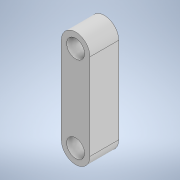
# Autodesk Inventor part: GearLock
Saved by Autodesk Inventor 2021 (Build 250183000, 183)
## iProperties
Created: 2021-03-28
Part Number: GearLock
Material: Generic
Document SubType Name: Modeling
Designer: elmar
Density: 1 g/cm^3
Appearance: Default
Author: elmar
Autodesk Inventor part; units mm, degrees
ref_plane "YZ Plane" through (0, 0, 0) normal (1, 0, 0) x (0, 1, 0)
ref_plane "XZ Plane" through (0, 0, 0) normal (0, 1, 0) x (-1, 0, 0)
ref_plane "XY Plane" through (0, 0, 0) normal (0, 0, 1) x (1, 0, 0)
sketch "Sketch1" plane through (0, 0, 0) normal (0, 0, 1) x (1, 0, 0)
  line L0 (0, -12) -> (0, 12) construction
  line L1 (4, -12) -> (4, 12)
  line L2 (-4, 12) -> (-4, -12)
  arc A0 (-4, -12) -> (4, -12) centre (0, -12) ccw
  arc A1 (4, 12) -> (-4, 12) centre (0, 12) ccw
  circle A2 centre (0, 12) radius 2.5
  circle A3 centre (0, -12) radius 2.5
  point P0 (0, 0)
  point P1 (0, 0)
  dimension "d0" = 24
  dimension "d1" = 8
  dimension "d2" = 5
  dimension "d3" = 5
  constraints: 8 end point, 4 centre point, 4 point on circle, 4 tangent, 3 coincident, 1 midpoint, 1 parallel, 1 vertical
  measures "d0" distance of L0.start L0.end
  measures "d1" distance between parallel lines of L1 L2
  measures "d2" diameter of A2
  measures "d3" diameter of A3
extrude "Extrusion1" add sketch "Sketch1" along normal blind 8
body "Solid1"
